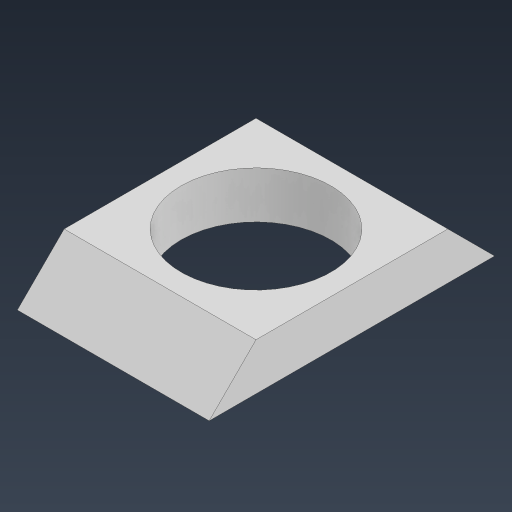
# Autodesk Inventor part: bearing_bed
Saved by Autodesk Inventor 2024 (Build 280153000, 153)
## iProperties
Created: 2024-10-09
Part Number: bearing_bed
Material: Generic
Document SubType Name: Modeling
Designer: Piter
Density: 1 g/cm^3
Appearance: Default
Author: Piter
Autodesk Inventor part; units mm, degrees
ref_plane "YZ Plane" through (0, 0, 0) normal (1, 0, 0) x (0, 1, 0)
ref_plane "XZ Plane" through (0, 0, 0) normal (0, 1, 0) x (-1, 0, 0)
ref_plane "XY Plane" through (0, 0, 0) normal (0, 0, 1) x (1, 0, 0)
sketch "Sketch1" plane through (0, 0, 0) normal (0, 1, 0) x (-1, 0, 0)
  line L0 (4.5242, 7.5266) -> (-15.9758, 7.5266)
  line L1 (-15.9758, 7.5266) -> (-15.9758, -12.9734)
  line L2 (-15.9758, -12.9734) -> (4.5242, -12.9734)
  line L3 (4.5242, -12.9734) -> (4.5242, 7.5266)
  circle A0 centre (-5.7258, -2.7234) radius 8
  point P0 (0, 0)
  dimension "d0" = 20.5
  dimension "d1" = 20.5
  dimension "d2" = 16
  constraints: 8 end point, 2 parallel, 1 centre point, 1 horizontal, 1 perpendicular
  measures "d0" distance of L2.end L1.end
  measures "d1" distance of L1.end L0.end
  measures "d2" diameter of A0
extrude "Extrusion1" add sketch "Sketch1" along normal blind 5
sketch "Sketch2" plane through (-4.5242, 0, -12.9734) normal (-1, 0, 0) x (0, 0, 1)
  line L0 (20.5, 0) -> (25.5, 0)
  line L1 (20.5, 0) -> (20.5, 5) projected
  line L2 (25.5, 0) -> (20.5, 5)
  line L3 (0, 0) -> (-5, 0)
  line L4 (-5, 0) -> (0, 5)
  line L5 (0, 0) -> (0, 5) projected
  line L6 (0, 5) -> (0, 0)
  point P0 (12.9734, 0)
  dimension "d6" = 5
  dimension "d7" = 5
  constraints: 10 end point, 2 horizontal, 1 vertical
  measures "d6" distance of L0.start L0.end
  measures "d7" distance of L3.start L3.end
extrude "Extrusion2" add sketch "Sketch2" against normal up to surface (20.5 mm away)
body "Solid1"
